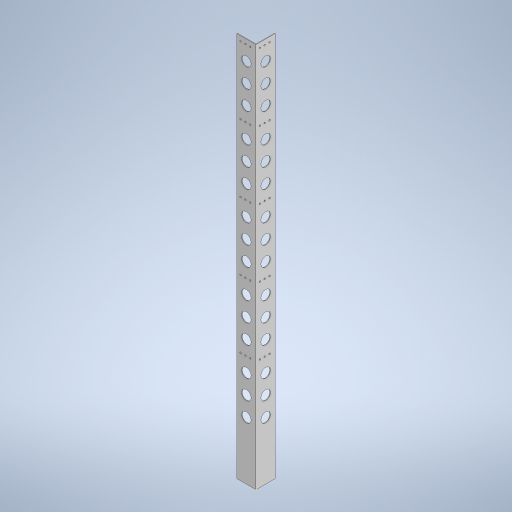
# Autodesk Inventor part: mesa completa
Saved by Autodesk Inventor 2024 (Build 280153000, 153)
## iProperties
Created: 2023-10-22
Part Number: mesa completa
Material: Genérico
Document SubType Name: Modeling
Designer: jhonc
Density: 1 g/cm^3
Appearance: Valor por defecto
Author: jhonc
Autodesk Inventor part; units mm, degrees
ref_plane "YZ Plane" through (0, 0, 0) normal (1, 0, 0) x (0, 1, 0)
ref_plane "XZ Plane" through (0, 0, 0) normal (0, 1, 0) x (-1, 0, 0)
ref_plane "XY Plane" through (0, 0, 0) normal (0, 0, 1) x (1, 0, 0)
sketch "Boceto6" plane through (0, 0, 0) normal (0, 1, 0) x (-1, 0, 0)
  line L0 (0, 0) -> (100, 0)
  line L1 (100, 0) -> (100, -100)
  line L2 (100, -100) -> (0, -100)
  line L3 (0, -100) -> (0, 0)
  line L4 (97, -97) -> (97, -3)
  line L5 (97, -3) -> (3, -3)
  line L6 (3, -3) -> (3, -97)
  line L7 (3, -97) -> (97, -97)
  line L8 (97, -3) -> (100, -3)
  line L9 (3, -97) -> (3, -106.6251)
  point P0 (3, -100)
  dimension "d46" = 100
  dimension "d47" = 100
  dimension "d48" = 3
  constraints: 20 end point, 4 parallel, 4 perpendicular, 1 horizontal, 1 point on line, 3 other
  measures "d46" distance of L0.start L0.end
  measures "d47" distance of L2.end L0.start
  measures "d48" distance between parallel lines of L1 L4
extrude "Extrusión6" add sketch "Boceto6" along normal blind 2000 contours L0 L1 L8 L5 L6 L9 L2 L3
sketch "Boceto9" plane through (-100, 0, 0) normal (0, 0, 1) x (1, 0, 0)
  point P0 (100, 0)
sketch "Boceto12" plane through (0, 0, 0) normal (1, 0, 0) x (0, 0, -1)
  line L0 (0, 2000) -> (100, 2000) projected
  line L1 (100, 0) -> (100, 2000) projected
  line L2 (0, 2000) -> (100, 2000)
  line L3 (100, 2000) -> (100, 1950)
  line L4 (100, 1950) -> (0, 1950)
  line L5 (0, 1950) -> (0, 2000)
  line L6 (0, 1650) -> (100, 1650)
  line L7 (100, 1650) -> (100, 1600)
  line L8 (100, 1600) -> (0, 1600)
  line L9 (0, 1600) -> (0, 1650)
  line L10 (0, 1300) -> (100, 1300)
  line L11 (100, 1300) -> (100, 1250)
  line L12 (100, 1250) -> (0, 1250)
  line L13 (0, 1250) -> (0, 1300)
  line L14 (0, 950) -> (100, 950)
  line L15 (100, 950) -> (100, 900)
  line L16 (100, 900) -> (0, 900)
  line L17 (0, 900) -> (0, 950)
  line L18 (0, 600) -> (100, 600)
  line L19 (100, 600) -> (100, 550)
  line L20 (100, 550) -> (0, 550)
  line L21 (0, 550) -> (0, 600)
  circle A0 centre (50, 1900) radius 25
  line L22 (0, 0) -> (0, 2000) projected
  circle A1 centre (50, 1800) radius 25
  circle A2 centre (50, 1700) radius 25
  circle A3 centre (20, 1975) radius 4
  circle A4 centre (45, 1975) radius 4
  circle A5 centre (70, 1975) radius 4
  line L23 (100, 1600) -> (0, 1600)
  line L24 (0, 1650) -> (100, 1650)
  line L25 (100, 1650) -> (100, 1600)
  circle A6 centre (50, 1350) radius 25
  circle A7 centre (50, 1450) radius 25
  circle A8 centre (50, 1550) radius 25
  circle A9 centre (70, 1625) radius 4
  circle A10 centre (45, 1625) radius 4
  circle A11 centre (20, 1625) radius 4
  line L26 (100, 1250) -> (0, 1250)
  line L27 (0, 1300) -> (100, 1300)
  line L28 (100, 1300) -> (100, 1250)
  circle A12 centre (50, 1000) radius 25
  circle A13 centre (50, 1100) radius 25
  circle A14 centre (50, 1200) radius 25
  circle A15 centre (70, 1275) radius 4
  circle A16 centre (45, 1275) radius 4
  circle A17 centre (20, 1275) radius 4
  line L29 (100, 900) -> (0, 900)
  line L30 (0, 950) -> (100, 950)
  line L31 (100, 950) -> (100, 900)
  circle A18 centre (50, 650) radius 25
  circle A19 centre (50, 750) radius 25
  circle A20 centre (50, 850) radius 25
  circle A21 centre (70, 925) radius 4
  circle A22 centre (45, 925) radius 4
  circle A23 centre (20, 925) radius 4
  line L32 (100, 550) -> (0, 550)
  line L33 (0, 600) -> (100, 600)
  line L34 (100, 600) -> (100, 550)
  circle A24 centre (50, 300) radius 25
  circle A25 centre (50, 400) radius 25
  circle A26 centre (50, 500) radius 25
  circle A27 centre (70, 575) radius 4
  circle A28 centre (45, 575) radius 4
  circle A29 centre (20, 575) radius 4
  point P0 (0, 1975)
  point P1 (100, 1975)
  point P2 (100, 1625)
  point P3 (100, 1275)
  point P4 (100, 925)
  point P5 (100, 575)
  dimension "d113" = 50
  dimension "d116" = 350
  dimension "d121" = 50
  dimension "d122" = 50
  dimension "d123" = 50
  dimension "d126" = 100
  dimension "d135" = 8
  dimension "d136" = 8
  dimension "d137" = 8
  dimension "d138" = 25
  dimension "d139" = 25
  dimension "d140" = 25
  dimension "d141" = 20
  dimension "d142" = 30
  dimension "d143" = 25
  dimension "d144" = 25
  dimension "d147" = 350
  constraints: 64 end point, 30 centre point, 2 equal radius, 2 midpoint, 2 parallel, 2 vertical, 2 vertical alignment, 1 horizontal, 1 perpendicular, 1 point on line, 113 other
  measures "d113" distance between parallel lines of L0 L4
  measures "d116" distance of L3.end L7.end
  measures "d121" diameter of A0
  measures "d122" distance from line of L4 A0.centre
  measures "d126" distance of A0.centre A1.centre
  measures "d135" diameter of A3
  measures "d136" diameter of A4
  measures "d137" diameter of A5
  measures "d138" distance from line of L0 A3.centre
  measures "d139" distance from line of L2 A4.centre
  measures "d140" distance from line of L0 A5.centre
  measures "d141" distance of A3.centre point (0, 1975)
  measures "d142" distance of point (100, 1975) A5.centre
  measures "d143" distance of A4.centre A3.centre
  measures "d144" distance of A5.centre A4.centre
  measures "d147" distance of L3.end L23.start
extrude "Extrusión10" cut sketch "Boceto12" against normal blind 2000 contours A0 | A1 | A2 | A3 | A4 | A5 | A6 | A7 | A8 | A9 | A10 | A11 | A12 | A13 | A14 | A15 | A16 | A17 | A18 | A19 | A20 | A21 | A22 | A23 | A24 | A25 | A26 | A27 | A28 | A29
sketch "Boceto13" plane through (-100, 0, 0) normal (0, 0, 1) x (1, 0, 0)
  line L0 (0, 2000) -> (100, 2000)
  line L1 (100, 694.7481) -> (100, 2000)
  line L2 (0, 2000) -> (100, 2000)
  line L3 (100, 2000) -> (100, 1950)
  line L4 (100, 1950) -> (0, 1950)
  line L5 (0, 1950) -> (0, 2000)
  line L6 (0, 1650) -> (100, 1650)
  line L7 (100, 1650) -> (100, 1600)
  line L8 (100, 1600) -> (0, 1600)
  line L9 (0, 1600) -> (0, 1650)
  line L10 (0, 1300) -> (100, 1300)
  line L11 (100, 1300) -> (100, 1250)
  line L12 (100, 1250) -> (0, 1250)
  line L13 (0, 1250) -> (0, 1300)
  line L14 (0, 950) -> (100, 950)
  line L15 (100, 950) -> (100, 900)
  line L16 (100, 900) -> (0, 900)
  line L17 (0, 900) -> (0, 950)
  line L18 (0, 600) -> (100, 600)
  line L19 (100, 600) -> (100, 550)
  line L20 (100, 550) -> (0, 550)
  line L21 (0, 550) -> (0, 600)
  circle A0 centre (50, 1900) radius 25
  line L22 (0, 692.1927) -> (0, 2000)
  circle A1 centre (50, 1800) radius 25
  circle A2 centre (50, 1700) radius 25
  circle A3 centre (20, 1975) radius 4
  circle A4 centre (45, 1975) radius 4
  circle A5 centre (70, 1975) radius 4
  line L23 (100, 1600) -> (0, 1600)
  line L24 (0, 1650) -> (100, 1650)
  line L25 (100, 1650) -> (100, 1600)
  circle A6 centre (50, 1350) radius 25
  circle A7 centre (50, 1450) radius 25
  circle A8 centre (50, 1550) radius 25
  circle A9 centre (70, 1625) radius 4
  circle A10 centre (45, 1625) radius 4
  circle A11 centre (20, 1625) radius 4
  line L26 (100, 1250) -> (0, 1250)
  line L27 (0, 1300) -> (100, 1300)
  line L28 (100, 1300) -> (100, 1250)
  circle A12 centre (50, 1000) radius 25
  circle A13 centre (50, 1100) radius 25
  circle A14 centre (50, 1200) radius 25
  circle A15 centre (70, 1275) radius 4
  circle A16 centre (45, 1275) radius 4
  circle A17 centre (20, 1275) radius 4
  line L29 (100, 900) -> (0, 900)
  line L30 (0, 950) -> (100, 950)
  line L31 (100, 950) -> (100, 900)
  circle A18 centre (50, 650) radius 25
  circle A19 centre (50, 750) radius 25
  circle A20 centre (50, 850) radius 25
  circle A21 centre (70, 925) radius 4
  circle A22 centre (45, 925) radius 4
  circle A23 centre (20, 925) radius 4
  line L32 (100, 550) -> (0, 550)
  line L33 (0, 600) -> (100, 600)
  line L34 (100, 600) -> (100, 550)
  circle A24 centre (50, 300) radius 25
  circle A25 centre (50, 400) radius 25
  circle A26 centre (50, 500) radius 25
  circle A27 centre (70, 575) radius 4
  circle A28 centre (45, 575) radius 4
  circle A29 centre (20, 575) radius 4
  line L35 (0, 0) -> (0, 2000) projected
  line L36 (100, 0) -> (100, 2000) projected
  line L37 (0, 2000) -> (100, 2000) projected
  point P0 (0, 1975)
  point P1 (100, 1975)
  point P2 (100, 1625)
  point P3 (100, 1275)
  point P4 (100, 925)
  point P5 (100, 575)
  dimension "d166" = 50
  dimension "d167" = 350
  dimension "d168" = 50
  dimension "d169" = 50
  dimension "d170" = 50
  dimension "d171" = 100
  dimension "d172" = 8
  dimension "d173" = 8
  dimension "d174" = 8
  dimension "d175" = 25
  dimension "d176" = 25
  dimension "d177" = 25
  dimension "d178" = 20
  dimension "d179" = 30
  dimension "d180" = 25
  dimension "d181" = 25
  dimension "d182" = 350
  dimension "d186" = 0
  dimension "d187" = 0
  dimension "d188" = 0
  constraints: 68 end point, 30 centre point, 2 equal radius, 2 midpoint, 2 parallel, 2 vertical, 2 vertical alignment, 1 horizontal, 1 perpendicular, 1 point on line, 115 other
  measures "d166" distance between parallel lines of L0 L4
  measures "d167" distance of L4.start L7.end
  measures "d168" diameter of A0
  measures "d169" distance from line of L4 A0.centre
  measures "d171" distance of A0.centre A1.centre
  measures "d172" diameter of A3
  measures "d173" diameter of A4
  measures "d174" diameter of A5
  measures "d175" distance from line of L0 A3.centre
  measures "d176" distance from line of L2 A4.centre
  measures "d177" distance from line of L0 A5.centre
  measures "d178" distance of A3.centre point (0, 1975)
  measures "d179" distance of point (100, 1975) A5.centre
  measures "d180" distance of A4.centre A3.centre
  measures "d181" distance of A5.centre A4.centre
  measures "d182" distance of L4.start L23.start
  measures "d186" horizontal extent of L35
  measures "d187" distance between parallel lines of L36 L1
  measures "d188" distance between parallel lines of L37 L0
extrude "Extrusión11" cut sketch "Boceto13" against normal blind 2000 contours A0 | A1 | A2 | A3 | A4 | A5 | A6 | A7 | A8 | A9 | A10 | A11 | A12 | A13 | A14 | A15 | A16 | A17 | A18 | A19 | A20 | A21 | A22 | A23 | A24 | A25 | A26 | A27 | A28 | A29
